honda_cup_holder_rail_v1 (Autodesk Fusion 360 design; units mm, degrees)
Autodesk Fusion 360 part; units mm, degrees
sketch "Rail Sketch" plane through (0, 0, 0) normal (1, 0, 0) x (0, 0, -1)
  line L0 (0, 0) -> (0, 10.4)
  line L1 (0, 10.4) -> (-11, 10.4)
  line L2 (-11, 0) -> (-16, 2.95)
  line L3 (-16, 7.45) -> (-11, 10.4)
  line L4 (-16, 2.95) -> (-16, 7.45)
  line L5 (-11, 0) -> (0, 0)
  dimension "d1" = 5
  dimension "d2" = 4.5
  dimension "d3" = 10.4
  dimension "d4" = 16
  constraint perpendicular L0 L1
  constraint perpendicular L0 L5
  constraint equal L1 L5
  constraint equal L2 L3
  constraint horizontal L1
  constraint coincident L0.end L1.start
  constraint coincident L0.start L5.end
  measures "d1" distance of L2.start L4
  measures "d2" distance of L2.end L3.start
  measures "d3" distance of L0.start L0.end
  measures "d4" distance of L0 L4
extrude "Extrude1" add sketch "Rail Sketch" along normal blind 15.5
sketch "Back Hole" plane through (0, 0, 0) normal (0, 0, -1) x (-1, 0, 0)
  line L0 (0, 0) -> (0, 10.4)
  line L1 (0, 10.4) -> (-15.5, 10.4)
  line L2 (-15.5, 10.4) -> (-15.5, 0)
  line L3 (-15.5, 0) -> (0, 0)
  line L4 (-14, 8.9) -> (-1.5, 8.9)
  line L5 (-1.5, 8.9) -> (-1.5, 1.5)
  line L6 (-1.5, 1.5) -> (-14, 1.5)
  line L7 (-14, 1.5) -> (-14, 8.9)
  dimension "d8" = 1.5
  dimension "d9" = 1.5
  dimension "d10" = 1.5
  dimension "d11" = 1.5
  constraint horizontal L4
  constraint vertical L5
  constraint horizontal L6
  constraint vertical L7
  measures "d8" distance of L2 L7
  measures "d9" distance of L1 L4 L6.end
  measures "d10" distance of L0 L5
  measures "d11" distance of L3 L6
extrude "Extrude2" cut sketch "Back Hole" against normal blind 11.5 contours L4 L5 L6 L7
sketch "Cross" plane through (0, 0, 11.5) normal (0, 0, -1) x (-1, 0, 0)
  line L0 (-14, 1.5) -> (-1.5, 1.5)
  line L1 (-1.5, 1.5) -> (-1.5, 8.9)
  line L2 (-1.5, 8.9) -> (-14, 8.9)
  line L3 (-14, 8.9) -> (-14, 1.5)
  line L4 (-7.75, 8.9) -> (-8.25, 8.9)
  line L5 (-8.25, 5.7) -> (-14, 5.7)
  line L6 (-14, 5.2) -> (-14, 4.7)
  line L7 (-8.25, 4.7) -> (-8.25, 1.5)
  line L8 (-7.75, 1.5) -> (-7.25, 1.5)
  line L9 (-7.25, 4.7) -> (-1.5, 4.7)
  line L10 (-1.5, 5.2) -> (-1.5, 5.7)
  line L11 (-14, 4.7) -> (-8.25, 4.7)
  line L12 (-7.25, 1.5) -> (-7.25, 1.6)
  line L13 (-7.25, 1.6) -> (-7.25, 4.7)
  line L14 (-1.5, 4.7) -> (-1.5, 5.2)
  line L15 (-1.5, 5.7) -> (-7.25, 5.7)
  line L16 (-7.25, 5.7) -> (-7.25, 8.9)
  line L17 (-7.75, 8.9) -> (-7.25, 8.9)
  line L18 (-8.25, 8.9) -> (-8.25, 5.7)
  line L19 (-8.25, 1.5) -> (-7.75, 1.5)
  line L20 (-14, 5.7) -> (-14, 5.2)
  dimension "d16" = 1
  constraint midpoint L2 L4.start
  constraint coincident L2 L4.end
  constraint parallel L2 L4
  constraint coincident L3 L5.end
  constraint perpendicular L3 L5
  constraint midpoint L3 L6.start
  constraint coincident L3 L6.end
  constraint perpendicular L5 L6
  constraint coincident L0 L7.end
  constraint perpendicular L0 L7
  constraint midpoint L0 L8.start
  constraint coincident L0 L8.end
  constraint perpendicular L7 L8
  constraint coincident L1 L9.end
  constraint perpendicular L1 L9
  constraint midpoint L1 L10.start
  constraint coincident L1 L10.end
  constraint perpendicular L9 L10
  constraint perpendicular L7 L11
  constraint perpendicular L8 L12
  constraint perpendicular L9 L13
  constraint perpendicular L1 L15
  constraint coincident L2 L16.end
  constraint perpendicular L2 L16
  constraint perpendicular L5 L18
  constraint equal L8 L19
  constraint collinear L13 L16
  constraint collinear L7 L18
  constraint collinear L5 L15
  constraint collinear L9 L11
  constraint equal L6 L20
  constraint equal L4 L20
  measures "d16" distance of L16 L18
extrude "Extrude3" add sketch "Cross" along normal blind 6.5 contours L0 L1 L2 L3 L4 L5 L6 L7 L8 L9 L10 L11 L12 L13 L14 L15 L16 L17 L18 L19 L20
sketch "Vertical Support" plane through (0, 0, 0) normal (0, 0, -1) x (-1, 0, 0)
  line L0 (-1.5, 8.9) -> (-1.5, 1.5)
  line L1 (-1.5, 1.5) -> (-14, 1.5)
  line L2 (-14, 1.5) -> (-14, 8.9)
  line L3 (-14, 8.9) -> (-1.5, 8.9)
  line L4 (0, 0) -> (0, 10.4)
  line L5 (0, 10.4) -> (-15.5, 10.4)
  line L6 (-15.5, 10.4) -> (-15.5, 0)
  line L7 (-15.5, 0) -> (0, 0)
  line L8 (-8.75, 10.4) -> (-7.75, 10.4)
  line L9 (-7.75, 10.4) -> (-6.75, 10.4)
  line L10 (-6.75, 12.9) -> (-6.75, 10.4)
  line L11 (-6.75, 12.9) -> (-8.75, 12.9)
  line L12 (-8.75, 12.9) -> (-8.75, 10.4)
  dimension "d19" = 2
  dimension "d20" = 2.5
  constraint coincident L5 L8.start
  constraint midpoint L5 L8.end
  constraint parallel L5 L8
  constraint coincident L5 L9.end
  constraint parallel L5 L9
  constraint perpendicular L9 L10
  constraint perpendicular L10 L11
  constraint vertical L12
  constraint equal L8 L9
  measures "d19" distance of L10.start L11.end
  measures "d20" distance of L9 L11
extrude "Extrude4" add sketch "Vertical Support" against normal blind 10.5 contours L5 L8 L9 L10 L11 L12
sketch "Right Fin " plane through (15.5, 0, 0) normal (1, 0, 0) x (0, 0, -1)
  line L0 (-16, 2.95) -> (-11, 0)
  line L1 (-11, 0) -> (0, 0)
  line L2 (0, 0) -> (0, 10.4)
  line L3 (0, 10.4) -> (-11, 10.4)
  line L4 (-11, 10.4) -> (-16, 7.45)
  line L5 (-16, 7.45) -> (-16, 2.95)
  line L6 (-1, 8.9) -> (-1, 1.5)
  line L7 (-1, 1.5) -> (-4, 1.5)
  line L8 (-4, 1.5) -> (-4, 8.9)
  line L9 (-4, 8.9) -> (-1, 8.9)
  dimension "d23" = 1.5
  dimension "d24" = 1.5
  dimension "d25" = 3
  dimension "d26" = 1
  constraint parallel L2 L6
  constraint perpendicular L6 L7
  constraint perpendicular L7 L8
  constraint perpendicular L6 L9
  measures "d23" distance of L3 L9
  measures "d24" distance of L1 L7
  measures "d25" distance of L6.start L8.end
  measures "d26" distance of L2 L6
extrude "Extrude5" add sketch "Right Fin " along normal blind 1.5 contours L6 L7 L8 L9
sketch "Right Fin Slice" plane through (0, 8.9, 0) normal (0, 1, 0) x (-1, 0, 0)
  line L0 (-15.5, 1) -> (-15.5, 4)
  line L1 (-15.5, 4) -> (-17, 4)
  line L2 (-17, 4) -> (-17, 1)
  line L3 (-17, 1) -> (-15.5, 1)
  line L4 (-15.5, 1) -> (-17, 4)
  constraint coincident L0.start L3.end
  constraint coincident L1.end L2.start
extrude "Extrude6" cut sketch "Right Fin Slice" against normal blind 7.4 contours L2 L3 L4
sketch "Left Fin" plane through (0, 0, 0) normal (-1, 0, 0) x (0, 0, 1)
  line L0 (11, 0) -> (16, 2.95)
  line L1 (16, 2.95) -> (16, 7.45)
  line L2 (16, 7.45) -> (11, 10.4)
  line L3 (11, 10.4) -> (0, 10.4)
  line L4 (0, 10.4) -> (0, 0)
  line L5 (0, 0) -> (11, 0)
  line L6 (1, 8.9) -> (4, 8.9)
  line L7 (4, 8.9) -> (4, 1.5)
  line L8 (4, 1.5) -> (1, 1.5)
  line L9 (1, 1.5) -> (1, 8.9)
  dimension "d31" = 1
  dimension "d32" = 3
  dimension "d33" = 1.5
  dimension "d34" = 1.5
  constraint horizontal L6
  constraint vertical L7
  constraint horizontal L8
  constraint vertical L9
  measures "d31" distance of L4 L9
  measures "d32" distance of L6.start L6.end
  measures "d33" distance of L3 L6
  measures "d34" distance of L5 L8
extrude "Extrude7" add sketch "Left Fin" along normal blind 1 contours L6 L7 L8 L9
sketch "Left Fin Slice" plane through (0, 8.9, 0) normal (0, 1, 0) x (-1, 0, 0)
  line L0 (0, 4) -> (0, 1)
  line L1 (0, 1) -> (1, 1)
  line L2 (1, 1) -> (1, 4)
  line L3 (1, 4) -> (0, 4)
  line L4 (0, 1) -> (1, 4)
  constraint coincident L0.end L1.start
  constraint coincident L2.end L3.start
extrude "Extrude8" cut sketch "Left Fin Slice" against normal blind 7.4 contours L1 L2 L4
equation "d17 = 11.5 mm - 5 mm"
